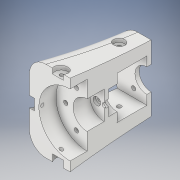
# Autodesk Inventor part: AA016
Saved by Autodesk Inventor 2017 SP1 (Build 210196100, 196)
## iProperties
Created: 2017-09-29
Part Number: AA016
Material: ABS Plastic
Document SubType Name: Modeling
Designer: Zach
Density: 1.06 g/cm^3
Appearance: CR White
Author: Zach
Autodesk Inventor part; units mm, degrees
ref_plane "XY Plane" through (0, 0, 0) normal (0, 0, 1) x (1, 0, 0)
sketch "Sketch1" plane through (0, 0, 0) normal (0, 0, 1) x (1, 0, 0)
  line L0 (0, 0) -> (70, 0)
  line L1 (70, 0) -> (70, 77.5)
  line L2 (70, 77.5) -> (0, 77.5)
  line L3 (0, 77.5) -> (0, 0)
  dimension "d0" = 70
  dimension "d1" = 77.5
  constraints: 8 end point, 2 parallel, 1 horizontal, 1 perpendicular
  measures "d0" distance of L2.end L1.end
  measures "d1" distance of L1.end L0.end
extrude "Extrusion1" add sketch "Sketch1" along normal blind 95
sketch "Sketch3" plane through (0, 0, 95) normal (0, 0, 1) x (1, 0, 0)
  line L0 (0, 0) -> (70, 0) projected
  line L1 (70, 77.5) -> (0, 77.5) projected
  line L2 (70, 0) -> (35, 0)
  line L3 (35, 0) -> (35, 77.5)
  line L4 (35, 77.5) -> (70, 77.5)
  line L5 (70, 77.5) -> (70, 0)
  constraints: 8 end point, 2 parallel, 1 horizontal, 1 midpoint, 1 perpendicular
extrude "Extrusion3" cut sketch "Sketch3" against normal through all
sketch "Sketch4" plane through (0, 77.5, 95) normal (0, 1, 0) x (1, 0, 0)
  line L0 (0, 95) -> (0, 0) projected
  line L1 (0, 0) -> (-12.5, 0)
  line L2 (35, 95) -> (0, 95) projected
  arc A0 (-12.5, 0) -> (0, 95) centre (-1145.4326, 197.3924) ccw
  line L3 (-12.5, -10) -> (35, -10) construction
  dimension "d9" = 1150
  dimension "d54" = 47.5
  dimension "d55" = 10
  constraints: 4 end point, 2 horizontal, 2 point on circle, 2 vertical alignment, 1 centre point
  measures "d9" radius of A0
  measures "d54" distance of L3.start L3.end
  measures "d55" distance between parallel lines of L1 L3
extrude "Extrusion4" add sketch "Sketch4" against normal blind 77.5
sketch "Sketch5" plane through (35, 0, 95) normal (1, 0, 0) x (0, 0, -1)
  line L0 (0, 77.5) -> (0, 86.25)
  line L1 (0, 0) -> (0, -8.75)
  line L2 (0, 0) -> (0, 77.5) projected
  line L3 (95, 77.5) -> (95, 0) projected
  arc A0 (0, 86.25) -> (95, 77.5) centre (152.8838, 1226.0423) ccw
  arc A1 (95, 0) -> (0, -8.75) centre (152.8838, -1148.5423) ccw
  line L4 (0, 77.5) -> (95, 77.5) projected
  line L5 (95, 0) -> (0, 0) projected
  line L6 (-10, 86.25) -> (-10, -8.75) construction
  point P0 (-10, 38.75)
  point P1 (0, 38.75)
  dimension "d14" = 1150
  dimension "d15" = 1150
  dimension "d52" = 10
  dimension "d53" = 95
  constraints: 6 end point, 4 point on circle, 3 horizontal alignment, 3 vertical, 2 centre point, 2 midpoint
  measures "d14" radius of A0
  measures "d15" radius of A1
  measures "d52" distance between parallel lines of L2 L6
  measures "d53" distance of L6.start L6.end
extrude "Extrusion5" add sketch "Sketch5" against normal blind 55 contours L0 A0 L4 | L5 A1 L1
sketch "Sketch6" plane through (-20, 0, 0) normal (0, 1, 0) x (1, 0, 0)
  line L0 (20, 0) -> (0, 0) projected
  line L1 (0, -95) -> (0, 0) projected
  arc A0 (7.5, -95) -> (20, 0) centre (-1125.4326, 102.3924) ccw projected
  line L2 (7.5, -95) -> (0, -95) projected
extrude "Extrusion6" cut sketch "Sketch6" along normal through all both and the other way through all
fillet "Fillet3" radius 19.35 2 edges at (-5.299, 80.9203, 47.9253) (-5.299, -3.4203, 47.9253)
sketch "Sketch8" plane through (0, 0, 95) normal (0, 0, 1) x (1, 0, 0)
  line L0 (35, 86.25) -> (35, -8.75) projected
  line L1 (35, 77.5) -> (35, 0) projected
  circle A0 centre (35, 38.75) radius 36.5
  point P0 (0, 0)
  dimension "d23" = 73
  constraints: 1 centre point, 1 midpoint
  measures "d23" diameter of A0
extrude "Extrusion7" cut sketch "Sketch8" against normal blind 20
sketch "Sketch9" plane through (0, 0, 75) normal (0, 0, 1) x (1, 0, 0)
  line L0 (35, 75.25) -> (35, 2.25) projected
  circle A0 centre (35, 38.75) radius 16.5
  point P0 (0, 0)
  dimension "d26" = 33
  constraints: 1 centre point, 1 midpoint
  measures "d26" diameter of A0
extrude "Extrusion8" cut sketch "Sketch9" against normal blind 20
sketch "Sketch10" plane through (0, 0, 0) normal (0, 0, -1) x (-1, 0, 0)
  line L0 (-35, 77.5) -> (-35, 0) projected
  circle A0 centre (-35, 38.75) radius 14
  point P0 (0, 0)
  dimension "d29" = 28
  constraints: 1 centre point, 1 midpoint
  measures "d29" diameter of A0
extrude "Extrusion9" cut sketch "Sketch10" against normal blind 50
sketch "Sketch11" plane through (0, 0, 50) normal (0, 0, -1) x (-1, 0, 0)
  line L0 (-35, 24.75) -> (-35, 52.75) projected
  circle A0 centre (-35, 38.75) radius 2.5
  circle A1 centre (-26.5, 38.75) radius 2
  point P0 (0, 0)
  dimension "d32" = 5
  dimension "d33" = 4
  dimension "d34" = 8.5
  constraints: 3 midpoint, 2 centre point, 2 horizontal alignment
  measures "d32" diameter of A0
  measures "d33" diameter of A1
  measures "d34" distance of A0.centre A1.centre
extrude "Extrusion10" cut sketch "Sketch11" against normal through all
sketch "Sketch12" plane through (0, 0, 55) normal (0, 0, 1) x (1, 0, 0)
  circle A0 centre (26.5, 38.75) radius 2 projected
  circle A1 centre (26.5, 38.75) radius 4.5
  point P0 (0, 0)
  dimension "d37" = 9
  constraints: 1 centre point, 1 coincident
  measures "d37" diameter of A1
extrude "Extrusion11" cut sketch "Sketch12" against normal blind 3
sketch "Sketch14" plane through (0, 0, 50) normal (0, 0, -1) x (-1, 0, 0)
  arc A0 (-35, 36.25) -> (-35, 41.25) centre (-35, 38.75) ccw projected
  circle A1 centre (-35, 38.75) radius 4
  point P0 (0, 0)
  dimension "d40" = 8
  constraints: 1 centre point, 1 coincident
  measures "d40" diameter of A1
extrude "Extrusion12" cut sketch "Sketch14" against normal blind 3
sketch "Sketch15" plane through (0, 0, 75) normal (0, 0, 1) x (1, 0, 0)
  arc A0 (35, 41.25) -> (35, 36.25) centre (35, 38.75) ccw projected
  circle A1 centre (10, 38.75) radius 2.5
  circle A2 centre (22.5, 17.0994) radius 2.5
  circle A3 centre (47.5, 17.0994) radius 2.5
  circle A4 centre (60, 38.75) radius 2.5
  circle A5 centre (47.5, 60.4006) radius 2.5
  circle A6 centre (22.5, 60.4006) radius 2.5
  point P0 (0, 0)
  dimension "d43" = 5
  dimension "d44" = 25
  dimension "d47" = 360
  constraints: 6 centre point, 1 horizontal alignment, 13 other
  measures "d43" diameter of A1
  measures "d44" distance of A0.centre A1.centre
extrude "Extrusion13" cut sketch "Sketch15" against normal blind 25
sketch "Sketch16" plane through (0, 0, 0) normal (0, 0, -1) x (-1, 0, 0)
  line L0 (-19.5, 54.25) -> (-19.5, 23.25) construction
  arc A0 (-35, 36.25) -> (-35, 41.25) centre (-35, 38.75) ccw projected
  circle A1 centre (-19.5, 23.25) radius 2.5
  circle A2 centre (-19.5, 54.25) radius 2.5
  line L1 (-35, 24.75) -> (-35, 0) projected
  point P0 (0, 0)
  point P1 (-19.5, 38.75)
  dimension "d56" = 31
  dimension "d57" = 5
  dimension "d58" = 5
  dimension "d59" = 15.5
  constraints: 2 centre point, 2 coincident, 2 end point, 1 horizontal alignment, 1 midpoint, 1 vertical
  measures "d56" distance of L0.start L0.end
  measures "d57" diameter of A1
  measures "d58" diameter of A2
  measures "d59" distance between parallel lines of L1 L0
extrude "Extrusion14" cut sketch "Sketch16" against normal blind 25
sketch "Sketch17" plane through (35, 75.25, 95) normal (1, 0, 0) x (0, 0, -1)
  line L0 (90, -61.5) -> (55, -61.5)
  line L1 (55, -61.5) -> (55, -11.5)
  line L2 (55, -11.5) -> (90, -11.5)
  line L3 (90, -11.5) -> (90, -61.5)
  line L4 (95, -22.5) -> (95, -50.5) projected
  point P0 (95, -75.25)
  point P1 (90, -36.5)
  point P2 (95, -36.5)
  dimension "d62" = 35
  dimension "d63" = 50
  dimension "d64" = 5
  constraints: 8 end point, 2 midpoint, 2 parallel, 1 horizontal, 1 horizontal alignment, 1 perpendicular
  measures "d62" distance of L1.end L2.end
  measures "d63" distance of L0.end L1.end
  measures "d64" distance from line of L3 point (95, -75.25)
extrude "Extrusion15" cut sketch "Sketch17" against normal through all
sketch "Sketch18" plane through (35, 63.75, 5) normal (0, -1, 0) x (1, 0, 0)
  circle A0 centre (-15, 17.5) radius 2.5
  line L0 (0, 0) -> (0, 35) projected
  point P0 (-35, -5)
  point P1 (0, 17.5)
  dimension "d67" = 5
  dimension "d68" = 15
  constraints: 1 centre point, 1 horizontal alignment, 1 midpoint
  measures "d67" diameter of A0
  measures "d68" distance of point (0, 17.5) A0.centre
extrude "Extrusion16" cut sketch "Sketch18" along normal through all both and the other way through all
ref_plane "Work Plane1" through (35, 86.25, 95) normal (0, 1, 0) x (-1, 0, 0)
sketch "Sketch19" plane through (35, 86.25, 95) normal (0, 1, 0) x (-1, 0, 0)
  spline S0 degree 8 poles (12.5, -72.5) (12.5, -72.1962) (12.5422, -71.9003) (12.6227, -71.6187) (12.7369, -71.3568) (12.8792, -71.1191) (13.0431, -70.9085) (13.2214, -70.7268) (13.5846, -70.4263) (13.7731, -70.3021) (13.9691, -70.2001) (14.1704, -70.1196) (14.3755, -70.0597) (14.5828, -70.0199) (14.7913, -70) (15.2604, -70) (15.5205, -70.031) (15.7784, -70.0929) (16.0318, -70.1863) (16.278, -70.3128) (16.5131, -70.4738) (16.7317, -70.6713) (17.0919, -71.1067) (17.2462, -71.3416) (17.3758, -71.6078) (17.4706, -71.8989) (17.524, -72.206) (17.5326, -72.5189) (17.497, -72.8273) (17.3726, -73.3119) (17.3067, -73.4977) (17.2242, -73.6773) (17.1258, -73.8491) (17.0123, -74.0112) (16.8849, -74.1624) (16.7448, -74.3011) (16.4271, -74.564) (16.2471, -74.6852) (16.0554, -74.7884) (15.8541, -74.8724) (15.6455, -74.936) (15.432, -74.9787) (15.216, -75) (14.7913, -75) (14.5828, -74.9801) (14.3755, -74.9403) (14.1705, -74.8804) (13.9691, -74.7999) (13.7731, -74.6979) (13.5846, -74.5737) (13.2215, -74.2733) (13.0431, -74.0916) (12.8792, -73.8809) (12.7369, -73.6431) (12.6227, -73.3811) (12.5421, -73.0995) (12.5, -72.8036) (12.5, -72.5) knots 0 0 0 0 0 0 0 0 0 0.142673 0.142673 0.142673 0.142673 0.142673 0.142673 0.142673 0.280066 0.280066 0.280066 0.280066 0.280066 0.280066 0.280066 0.451558 0.451558 0.451558 0.451558 0.451558 0.451558 0.451558 0.597583 0.597583 0.597583 0.597583 0.597583 0.597583 0.597583 0.691916 0.691916 0.691916 0.691916 0.691916 0.691916 0.691916 0.795687 0.795687 0.795687 0.795687 0.795687 0.795687 0.795687 0.895946 0.895946 0.895946 0.895946 0.895946 0.895946 0.895946 1 1 1 1 1 1 1 1 1 projected
  circle A0 centre (15, -72.5) radius 2.5 projected
  circle A1 centre (15, -72.5) radius 6.5
  point P0 (35, -95)
  dimension "d71" = 13
  constraints: 1 centre point, 1 coincident, 1 vertical alignment, 1 other
  measures "d71" diameter of A1
extrude "Extrusion17" cut sketch "Sketch19" against normal blind 12
ref_plane "Work Plane2" through (35, -8.75, 95) normal (0, 1, 0) x (-1, 0, 0)
sketch "Sketch20" plane through (35, -8.75, 95) normal (0, 1, 0) x (-1, 0, 0)
  spline S0 degree 8 poles (12.5, -72.5) (12.5, -72.1962) (12.5422, -71.9003) (12.6227, -71.6187) (12.7369, -71.3568) (12.8792, -71.1191) (13.0431, -70.9085) (13.2214, -70.7268) (13.5846, -70.4263) (13.7731, -70.3021) (13.9691, -70.2001) (14.1704, -70.1196) (14.3755, -70.0597) (14.5828, -70.0199) (14.7913, -70) (15.2604, -70) (15.5205, -70.031) (15.7784, -70.0929) (16.0318, -70.1863) (16.278, -70.3128) (16.5131, -70.4738) (16.7317, -70.6713) (17.0919, -71.1067) (17.2462, -71.3416) (17.3758, -71.6078) (17.4706, -71.8989) (17.524, -72.206) (17.5326, -72.5189) (17.497, -72.8273) (17.3726, -73.3119) (17.3067, -73.4977) (17.2242, -73.6773) (17.1258, -73.8491) (17.0123, -74.0112) (16.8849, -74.1624) (16.7448, -74.3011) (16.4271, -74.564) (16.2471, -74.6852) (16.0554, -74.7884) (15.8541, -74.8724) (15.6455, -74.936) (15.432, -74.9787) (15.216, -75) (14.7913, -75) (14.5828, -74.9801) (14.3755, -74.9403) (14.1705, -74.8804) (13.9691, -74.7999) (13.7731, -74.6979) (13.5846, -74.5737) (13.2215, -74.2733) (13.0431, -74.0916) (12.8792, -73.8809) (12.7369, -73.6431) (12.6227, -73.3811) (12.5421, -73.0995) (12.5, -72.8036) (12.5, -72.5) knots 0 0 0 0 0 0 0 0 0 0.142673 0.142673 0.142673 0.142673 0.142673 0.142673 0.142673 0.280066 0.280066 0.280066 0.280066 0.280066 0.280066 0.280066 0.451558 0.451558 0.451558 0.451558 0.451558 0.451558 0.451558 0.597583 0.597583 0.597583 0.597583 0.597583 0.597583 0.597583 0.691916 0.691916 0.691916 0.691916 0.691916 0.691916 0.691916 0.795687 0.795687 0.795687 0.795687 0.795687 0.795687 0.795687 0.895946 0.895946 0.895946 0.895946 0.895946 0.895946 0.895946 1 1 1 1 1 1 1 1 1 projected
  circle A0 centre (15, -72.5) radius 6.5
  circle A1 centre (15, -72.5) radius 2.5 projected
  point P0 (35, -95)
  dimension "d74" = 13
  constraints: 1 centre point, 1 vertical alignment, 2 other
  measures "d74" diameter of A0
extrude "Extrusion18" cut sketch "Sketch20" along normal blind 12
sketch "Sketch21" plane through (35, 86.25, 95) normal (0, 1, 0) x (-1, 0, 0)
  circle A0 centre (14.1535, -4) radius 2
  line L0 (0, 0) -> (28.3069, 0) projected
  point P0 (35, -95)
  point P1 (14.1535, 0)
  dimension "d77" = 4
  dimension "d78" = 4
  constraints: 1 centre point, 1 midpoint, 1 vertical alignment
  measures "d77" diameter of A0
  measures "d78" distance from line of L0 A0.centre
extrude "Extrusion19" cut sketch "Sketch21" against normal through all
sketch "Sketch22" plane through (35, 86.25, 95) normal (0, 1, 0) x (-1, 0, 0)
  spline S0 degree 7 poles (16.1535, -4) (16.1535, -3.7251) (16.1094, -3.4575) (16.0254, -3.2053) (15.9073, -2.9753) (15.7625, -2.7728) (15.5995, -2.6006) (15.2664, -2.325) (15.093, -2.215) (14.9117, -2.1282) (14.7252, -2.0639) (14.5356, -2.0213) (14.3445, -2) (13.9146, -2) (13.6758, -2.0333) (13.44, -2.0998) (13.2105, -2.2006) (12.9915, -2.3372) (12.789, -2.5117) (12.459, -2.9106) (12.3197, -3.1321) (12.2104, -3.3851) (12.1422, -3.6607) (12.121, -3.9464) (12.1475, -4.2292) (12.261, -4.6713) (12.3238, -4.8405) (12.4043, -5.0027) (12.5014, -5.1558) (12.614, -5.2977) (12.7403, -5.4266) (13.0308, -5.6669) (13.1974, -5.7753) (13.3762, -5.8641) (13.5642, -5.9318) (13.7585, -5.9773) (13.956, -6) (14.3446, -6) (14.5357, -5.9787) (14.7253, -5.9361) (14.9116, -5.8718) (15.0928, -5.7851) (15.2662, -5.6751) (15.5994, -5.3995) (15.7624, -5.2273) (15.9074, -5.0247) (16.0255, -4.7946) (16.1095, -4.5423) (16.1535, -4.2747) (16.1535, -4) knots 0 0 0 0 0 0 0 0 0.142563 0.142563 0.142563 0.142563 0.142563 0.142563 0.277409 0.277409 0.277409 0.277409 0.277409 0.277409 0.446033 0.446033 0.446033 0.446033 0.446033 0.446033 0.592532 0.592532 0.592532 0.592532 0.592532 0.592532 0.687529 0.687529 0.687529 0.687529 0.687529 0.687529 0.792031 0.792031 0.792031 0.792031 0.792031 0.792031 0.893203 0.893203 0.893203 0.893203 0.893203 0.893203 1 1 1 1 1 1 1 1 projected
  circle A0 centre (14.1535, -4) radius 7.5
  line L0 (0, 0) -> (28.3069, 0) projected
  point P0 (35, -95)
  point P1 (14.1535, 0)
  dimension "d81" = 15
  dimension "d82" = 4
  constraints: 1 centre point, 1 midpoint, 1 vertical alignment, 1 other
  measures "d81" diameter of A0
  measures "d82" distance from line of A0.centre L0
extrude "Extrusion20" cut sketch "Sketch22" against normal blind 6
sketch "Sketch23" plane through (35, -8.75, 95) normal (0, 1, 0) x (-1, 0, 0)
  circle A0 centre (14.1535, -4) radius 2 projected
  circle A1 centre (14.1535, -4) radius 7.5
  point P0 (35, -95)
  dimension "d85" = 15
  constraints: 1 centre point, 1 coincident
  measures "d85" diameter of A1
extrude "Extrusion21" cut sketch "Sketch23" along normal blind 8
ref_plane "Work Plane3" through (-12.5, 38.75, 95) normal (-1, 0, 0) x (0, -1, 0)
sketch "Sketch24" plane through (-12.5, 38.75, 95) normal (-1, 0, 0) x (0, -1, 0)
  circle A0 centre (0, -4) radius 7.5
  line L0 (-28.4225, 0) -> (28.4225, 0) projected
  point P0 (38.75, -95)
  point P1 (0, 0)
  dimension "d88" = 15
  dimension "d89" = 4
  constraints: 1 centre point, 1 midpoint, 1 vertical alignment
  measures "d88" diameter of A0
  measures "d89" distance of point (0, 0) A0.centre
extrude "Extrusion22" cut sketch "Sketch24" against normal blind 6
sketch "Sketch25" plane through (-6.5, 38.75, 95) normal (-1, 0, 0) x (0, 0, 1)
  circle A0 centre (-4, 0) radius 2
  arc A1 (0, 6.3443) -> (0, -6.3443) centre (-4, 0) ccw projected
  point P0 (-95, -38.75)
  dimension "d92" = 4
  constraints: 1 centre point, 1 concentric
  measures "d92" diameter of A0
extrude "Extrusion23" cut sketch "Sketch25" against normal through all
body "Solid1"
